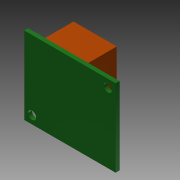
# Autodesk Inventor part: Driver Kipas v2
Saved by Autodesk Inventor 2015 (Build 190159000, 159)
## iProperties
Created: 2015-02-04
Part Number: Driver Kipas v2
Material: Generic
Document SubType Name: Modeling
Designer: Rafi Kurnia Putra
Density: 1 g/cm^3
Appearance: Smooth - Dark Forest Green
Mass: 6.77254 g
Surface Area: 39.979 cm^2
Volume: 6.77254 cm^3
Author: Rafi Kurnia Putra
Autodesk Inventor part; units mm, degrees
ref_plane "YZ Plane" through (0, 0, 0) normal (1, 0, 0) x (0, 1, 0)
ref_plane "XZ Plane" through (0, 0, 0) normal (0, 1, 0) x (-1, 0, 0)
ref_plane "XY Plane" through (0, 0, 0) normal (0, 0, 1) x (1, 0, 0)
sketch "Sketch1" plane through (0, 0, 0) normal (0, 1, 0) x (-1, 0, 0)
  line L0 (19.8755, 16.8275) -> (-19.8755, 16.8275)
  line L1 (-19.8755, 16.8275) -> (-19.8755, -16.8275)
  line L2 (-19.8755, -16.8275) -> (19.8755, -16.8275)
  line L3 (19.8755, -16.8275) -> (19.8755, 16.8275)
  line L4 (19.8755, 16.8275) -> (-19.8755, -16.8275) construction
  line L5 (-19.8755, 16.8275) -> (19.8755, -16.8275) construction
  circle A0 centre (16.4465, -13.3985) radius 1.75
  circle A1 centre (-16.4465, 13.3985) radius 1.75
  line L6 (15.8555, -1.8383) -> (-2.9345, -1.8383)
  line L7 (-2.9345, -1.8383) -> (-2.9345, 13.4817)
  line L8 (-2.9345, 13.4817) -> (15.8555, 13.4817)
  line L9 (15.8555, 13.4817) -> (15.8555, -1.8383)
  point P0 (0, 0)
  dimension "d0" = 39.751
  dimension "d1" = 33.655
  dimension "d2" = 3.5
  dimension "d3" = 3.5
  dimension "d4" = 3.429
  dimension "d5" = 3.429
  dimension "d6" = 3.429
  dimension "d7" = 3.429
  dimension "d8" = 18.79
  dimension "d9" = 15.32
  dimension "d10" = 24.2439
  dimension "d11" = 24.2439
  constraints: 20 end point, 4 parallel, 2 centre point, 2 horizontal, 2 midpoint, 2 perpendicular
  measures "d0" distance of L2.end L1.end
  measures "d1" distance of L1.end L0.end
  measures "d2" diameter of A0
  measures "d3" diameter of A1
  measures "d4" distance from line of A0.centre L3
  measures "d5" distance from line of L2 A0.centre
  measures "d6" distance from line of L1 A1.centre
  measures "d7" distance from line of A1.centre L0
  measures "d8" distance of L7.end L9.start
  measures "d9" distance of L7.start L7.end
  measures "d10" distance of L6.start L7.end
  measures "d11" distance of L9.start L7.start
extrude "Extrusion1" add sketch "Sketch1" along normal blind 1.7
extrude "Extrusion2" add sketch "Sketch1" along normal blind 17.44 contours L6 L7 L8 L9
sketch "Sketch2" plane through (0, 1.7, 0) normal (0, 1, 0) x (1, 0, 0)
  line L0 (-18.4674, 8.6665) -> (19.4938, 8.6665) construction
  line L1 (19.4938, 8.6665) -> (19.4938, 5.0304) construction
  line L2 (19.4938, 5.0304) -> (-18.4674, 5.0304) construction
  line L3 (-18.4674, 5.0304) -> (-18.4674, 8.6665) construction
  point P0 (0, 0)
  constraints: 2 other
body "Solid1"
